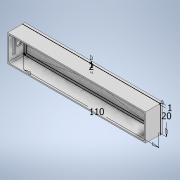
# Autodesk Inventor part: sdm_finger_bone_attachment_mould
Saved by Autodesk Inventor 2021 (Build 250183000, 183)
## iProperties
Created: 2021-05-26
Part Number: sdm_finger_bone_attachment_mould
Material: Generic
Document SubType Name: Modeling
Designer: Charlie
Density: 1 g/cm^3
Appearance: Default
Author: Charlie
Autodesk Inventor part; units mm, degrees
ref_plane "YZ Plane" through (0, 0, 0) normal (1, 0, 0) x (0, 1, 0)
ref_plane "XZ Plane" through (0, 0, 0) normal (0, 1, 0) x (-1, 0, 0)
ref_plane "XY Plane" through (0, 0, 0) normal (0, 0, 1) x (1, 0, 0)
sketch "Sketch2" plane through (0, 0, 0) normal (0, 0, 1) x (1, 0, 0)
  line L0 (-54, 10) -> (54, 10)
  line L1 (55, 9) -> (55, -9)
  line L2 (54, -10) -> (-54, -10)
  line L3 (-55, -9) -> (-55, 9)
  line L4 (-55, 10) -> (55, -10) construction
  line L5 (55, 10) -> (-55, -10) construction
  line L6 (53, 8) -> (-53, 8)
  line L7 (-53, 8) -> (-53, -8)
  line L8 (-53, -8) -> (53, -8)
  line L9 (53, -8) -> (53, 8)
  line L10 (56, 11) -> (-56, 11)
  line L11 (-56, 11) -> (-56, -11)
  line L12 (-56, -11) -> (56, -11)
  line L13 (56, -11) -> (56, 11)
  arc A0 (55, 9) -> (54, 10) centre (54, 9) ccw
  arc A1 (54, -10) -> (55, -9) centre (54, -9) ccw
  arc A2 (-55, -9) -> (-54, -10) centre (-54, -9) ccw
  arc A3 (-54, 10) -> (-55, 9) centre (-54, 9) ccw
  point P0 (0, 0)
  dimension "d0" = 110
  dimension "d1" = 20
  dimension "d2" = 2
  dimension "d3" = 1
  dimension "d10" = 1
  constraints: 28 end point, 8 point on circle, 8 point on line, 8 tangent, 6 parallel, 4 centre point, 3 equal radius, 3 perpendicular, 2 midpoint, 1 horizontal, 6 other
  measures "d0" distance of L4.end L5.end
  measures "d1" distance of L5.start L4.end
  measures "d2" distance between parallel lines of L0 L6
  measures "d3" distance between parallel lines of L0 L10
  measures "d10" radius of A0
extrude "Extrusion2" add sketch "Sketch2" along normal blind 12 contours L13 L12 L11 L10
sketch "Sketch3" plane through (-56, -11, 0) normal (-1, 0, 0) x (0, 0, 1)
  line L0 (7, 17) -> (9, 17)
  line L1 (9, 17) -> (9, 5)
  line L2 (9, 5) -> (7, 5)
  line L3 (7, 5) -> (7, 17)
  line L4 (0, 22) -> (0, 0) projected
  line L5 (0, 22) -> (12, 22) projected
  circle A0 centre (4, 11) radius 2
  line L6 (12, 22) -> (12, 0) projected
  line L7 (0, 11) -> (2, 11) construction
  dimension "d20" = 4
  dimension "d12" = 2
  dimension "d13" = 12
  dimension "d15" = 5
  dimension "d21" = 3
  dimension "d24" = 4
  dimension "d25" = 2
  dimension "d26" = 3
  constraints: 10 end point, 2 parallel, 1 horizontal, 1 horizontal alignment, 1 perpendicular, 2 other
  measures "d12" distance of L1.end L2.end
  measures "d13" distance of L0.end L1.end
  measures "d15" distance between parallel lines of L5 L0
  measures "d21" distance from line of L3 point (4, 11)
  measures "d24" distance from line of L4 point (4, 11)
  measures "d25" distance of L7.start L7.end
  measures "d26" distance between parallel lines of L6 L1
extrude "Extrusion4" cut sketch "Sketch3" against normal blind 10
extrude "Extrusion5" add sketch "Sketch2" against normal blind 2 contours L0 A0 L1 A1 L2 A2 L3 A3 | L9 L8 L7 L6 | L13 L12 L11 L10
body "Solid1"
